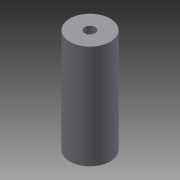
# Autodesk Inventor part: entretoise
Saved by Autodesk Inventor 2013 (Build 170138000, 138)
## iProperties
Created: 2013-06-25
Part Number: entretoise
Material: Generic
Document SubType Name: Modeling
Designer: Piotr
Density: 1 g/cm^3
Mass: 2.38826 g
Surface Area: 18.8068 cm^2
Volume: 2.38826 cm^3
Author: Piotr
Autodesk Inventor part; units mm, degrees
ref_plane "YZ Plane" through (0, 0, 0) normal (1, 0, 0) x (0, 1, 0)
ref_plane "XZ Plane" through (0, 0, 0) normal (0, 1, 0) x (-1, 0, 0)
ref_plane "XY Plane" through (0, 0, 0) normal (0, 0, 1) x (1, 0, 0)
sketch "Sketch1" plane through (0, 0, 0) normal (0, 0, 1) x (1, 0, 0)
  circle A0 centre (0, 0) radius 5.85
  dimension "d0" = 11.7
  constraints: 1 centre point, 1 coincident
  measures "d0" diameter of A0
extrude "Extrusion1" add sketch "Sketch1" along normal blind 30
hole "Hole1" at (0, 0, 0) direction (0, 0, 1) diameter 3.1 end through all
body "Solid1"
